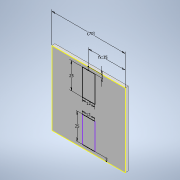
# Autodesk Inventor part: body
Saved by Autodesk Inventor 2022.2 (Build 262287010, 287A)
## iProperties
Created: 2022-02-20
Part Number: body
Material: Generic
Document SubType Name: Modeling
Designer: Nakai
Density: 1 g/cm^3
Appearance: Default
Author: Nakai
Autodesk Inventor part; units mm, degrees
ref_plane "YZ Plane" through (0, 0, 0) normal (1, 0, 0) x (0, 1, 0)
ref_plane "XZ Plane" through (0, 0, 0) normal (0, 1, 0) x (-1, 0, 0)
ref_plane "XY Plane" through (0, 0, 0) normal (0, 0, 1) x (1, 0, 0)
sketch "Sketch1" plane through (0, 0, 0) normal (0, 0, 1) x (1, 0, 0)
  line L0 (0, 0) -> (70, 0)
  line L1 (70, 0) -> (70, 70)
  line L2 (70, 70) -> (0, 70)
  line L3 (0, 70) -> (0, 0)
  dimension "d0" = 70
  dimension "d1" = 70
  constraints: 8 end point, 2 parallel, 1 horizontal, 1 perpendicular
  measures "d0" distance of L2.end L1.end
  measures "d1" distance of L1.end L0.end
extrude "Extrusion1" add sketch "Sketch1" along normal blind 3
sketch "Esboço3" plane through (0, 0, 3) normal (0, 0, 1) x (1, 0, 0)
  line L0 (70, 70) -> (0, 70) projected
  line L1 (70, 0) -> (70, 70) projected
  line L2 (0, 70) -> (0, 0) projected
  line L3 (41, 67) -> (29, 67)
  line L4 (29, 67) -> (29, 42)
  line L5 (29, 42) -> (41, 42)
  line L6 (41, 42) -> (41, 67)
  line L7 (41, 3) -> (29, 3)
  line L8 (29, 3) -> (29, 28)
  line L9 (29, 28) -> (41, 28)
  line L10 (41, 28) -> (41, 3)
  line L11 (0, 0) -> (70, 0) projected
  point P0 (35, 70)
  point P1 (35, 67)
  dimension "d10" = 70
  dimension "d11" = 12
  dimension "d12" = 25
  dimension "d13" = 3
  dimension "d14" = 35
  dimension "d15" = 12
  dimension "d16" = 25
  dimension "d17" = 3
  constraints: 16 end point, 4 parallel, 2 horizontal, 2 midpoint, 2 perpendicular
  measures "d10" distance between parallel lines of L2 L1
  measures "d11" distance of L5.end L4.end
  measures "d12" distance of L4.end L3.end
  measures "d13" distance from line of point (35, 70) L3
  measures "d14" distance from line of point (35, 67) L1
  measures "d15" distance of L8.end L9.end
  measures "d16" distance of L7.end L8.end
  measures "d17" distance between parallel lines of L11 L7
equation "\"d14\" = 0.5 * d10"
body "Solid1"
